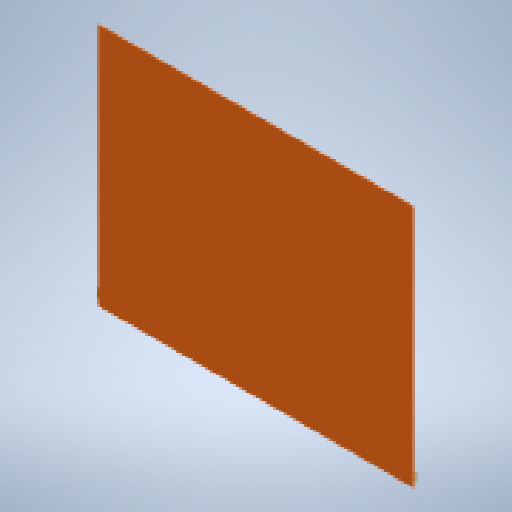
# Autodesk Inventor part: paperbodyfront
Saved by Autodesk Inventor 2025 (Build 290162000, 162)
## iProperties
Created: 2024-09-08
Part Number: paperbodyfront
Material: Generic
Document SubType Name: Modeling
Designer: Win
Density: 1 g/cm^3
Appearance: Smooth - Light Orange
Author: Win
Autodesk Inventor part; units mm, degrees
ref_plane "YZ Plane" through (0, 0, 0) normal (1, 0, 0) x (0, 1, 0)
ref_plane "XZ Plane" through (0, 0, 0) normal (0, 1, 0) x (-1, 0, 0)
ref_plane "XY Plane" through (0, 0, 0) normal (0, 0, 1) x (1, 0, 0)
ref_plane "Work Plane1" through (0, 2032, -1859.2927) normal (0, 0, 1) x (1, 0, 0)
sketch "Sketch1" plane through (0, 2032, -1859.2927) normal (0, 0, 1) x (1, 0, 0)
  line L0 (203.2, -50.8) -> (2438.4, -50.8) projected
  line L1 (203.2, -50.8) -> (101.6, -50.8) projected
  line L2 (101.6, -50.8) -> (101.6, 0) projected
  line L3 (101.6, 0) -> (101.6, 50.8) projected
  line L4 (101.6, 50.8) -> (101.6, 1727.2) projected
  line L5 (101.6, 1828.8) -> (101.6, 1727.2) projected
  line L6 (101.6, 1828.8) -> (2540, 1828.8) projected
  line L7 (2540, 1828.8) -> (2540, 1727.2) projected
  line L8 (2540, 50.8) -> (2540, 1727.2) projected
  line L9 (2540, 50.8) -> (2540, 0) projected
  line L10 (2540, 0) -> (2540, -50.8) projected
  line L11 (2540, -50.8) -> (2438.4, -50.8) projected
  point P0 (0, -2032)
  point P1 (101.6, 1727.2)
  point P2 (101.6, 50.8)
extrude "Extrusion1" add sketch "Sketch1" along normal blind 6.35
body "Solid1"
